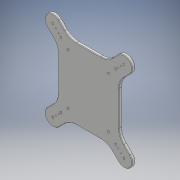
# Autodesk Inventor part: body
Saved by Autodesk Inventor 2018 (Build 220112000, 112)
## iProperties
Created: 2018-04-07
Part Number: body
Material: Generic
Document SubType Name: Modeling
Designer: Matyi
Density: 1 g/cm^3
Appearance: Default
Author: Matyi
Autodesk Inventor part; units mm, degrees
ref_plane "YZ Plane" through (0, 0, 0) normal (1, 0, 0) x (0, 1, 0)
ref_plane "XZ Plane" through (0, 0, 0) normal (0, 1, 0) x (-1, 0, 0)
ref_plane "XY Plane" through (0, 0, 0) normal (0, 0, 1) x (1, 0, 0)
sketch "Sketch1" plane through (0, 0, 0) normal (0, 1, 0) x (-1, 0, 0)
  line L0 (0, 0) -> (60, 0)
  line L1 (60, 0) -> (60, -70)
  line L2 (60, -70) -> (0, -70)
  line L3 (0, -70) -> (0, 0)
  circle A0 centre (3, -3) radius 1
  circle A1 centre (57, -3) radius 1
  circle A2 centre (57, -67) radius 1
  circle A3 centre (3, -67) radius 1
  circle A4 centre (65, 5) radius 1
  circle A5 centre (65, -75) radius 1
  circle A6 centre (-5, -75) radius 1
  circle A7 centre (-5, 5) radius 1
  arc A8 (0.6569, 10.6569) -> (-10.6569, -0.6569) centre (-5, 5) ccw
  line L4 (-5, 5) -> (0.6569, 10.6569) construction
  line L5 (-5, 5) -> (3, 5) construction
  line L6 (-5, 5) -> (-10.6569, -0.6569) construction
  arc A9 (70.6569, -0.6569) -> (59.3431, 10.6569) centre (65, 5) ccw
  line L7 (65, 5) -> (70.6569, -0.6569) construction
  line L8 (65, 5) -> (73, 5) construction
  line L9 (65, 5) -> (59.3431, 10.6569) construction
  arc A10 (59.3431, -80.6569) -> (70.6569, -69.3431) centre (65, -75) ccw
  line L10 (65, -75) -> (59.3431, -80.6569) construction
  line L11 (65, -75) -> (73, -75) construction
  line L12 (65, -75) -> (70.6569, -69.3431) construction
  arc A11 (-10.6569, -69.3431) -> (0.6569, -80.6569) centre (-5, -75) ccw
  line L13 (-5, -75) -> (0.6569, -80.6569) construction
  line L14 (-5, -75) -> (3, -75) construction
  line L15 (-5, -75) -> (-10.6569, -69.3431) construction
  line L16 (70.6569, -0.6569) -> (60, -11.3137)
  line L17 (59.3431, 10.6569) -> (48.6863, 0)
  line L18 (0.6569, 10.6569) -> (11.3137, 0)
  line L19 (-10.6569, -0.6569) -> (0, -11.3137)
  line L20 (-10.6569, -69.3431) -> (0, -58.6863)
  line L21 (0.6569, -80.6569) -> (11.3137, -70)
  line L22 (59.3431, -80.6569) -> (48.6863, -70)
  line L23 (70.6569, -69.3431) -> (60, -58.6863)
  circle A12 centre (62.1716, 2.1716) radius 0.5
  circle A13 centre (59.3431, -0.6569) radius 0.5
  line L24 (65, 5) -> (62.1716, 2.1716)
  line L25 (65, 5) -> (69, 5) construction
  line L26 (62.1716, 2.1716) -> (59.3431, -0.6569)
  line L27 (-5, 5) -> (-2.1716, 2.1716)
  line L28 (-2.1716, 2.1716) -> (0.6569, -0.6569)
  circle A14 centre (0.6569, -0.6569) radius 0.5
  circle A15 centre (-2.1716, 2.1716) radius 0.5
  line L29 (-5, -75) -> (-2.1716, -72.1716)
  line L30 (-2.1716, -72.1716) -> (0.6569, -69.3431)
  circle A16 centre (0.6569, -69.3431) radius 0.5
  circle A17 centre (-2.1716, -72.1716) radius 0.5
  line L31 (65, -75) -> (62.1716, -72.1716)
  line L32 (62.1716, -72.1716) -> (59.3431, -69.3431)
  circle A18 centre (59.3431, -69.3431) radius 0.5
  circle A19 centre (62.1716, -72.1716) radius 0.5
  circle A20 centre (50, -10) radius 1
  circle A21 centre (10, -10) radius 1
  circle A22 centre (50, -60) radius 1
  circle A23 centre (10, -60) radius 1
  dimension "d0" = 60
  dimension "d1" = 70
  dimension "d2" = 2
  dimension "d3" = 2
  dimension "d4" = 2
  dimension "d5" = 2
  dimension "d6" = 3
  dimension "d7" = 3
  dimension "d8" = 3
  dimension "d9" = 3
  dimension "d10" = 3
  dimension "d11" = 3
  dimension "d12" = 3
  dimension "d13" = 3
  dimension "d19" = 2
  dimension "d20" = 2
  dimension "d21" = 2
  dimension "d22" = 2
  dimension "d23" = 5
  dimension "d24" = 5
  dimension "d25" = 5
  dimension "d26" = 5
  dimension "d27" = 5
  dimension "d28" = 5
  dimension "d29" = 5
  dimension "d30" = 5
  dimension "d32" = 8
  dimension "d33" = 45
  dimension "d34" = 180
  dimension "d35" = 8
  dimension "d36" = 45
  dimension "d37" = 180
  dimension "d38" = 8
  dimension "d39" = 135
  dimension "d40" = 180
  dimension "d41" = 8
  dimension "d42" = 45
  dimension "d43" = 180
  dimension "d48" = 1
  dimension "d49" = 1
  dimension "d50" = 4
  dimension "d51" = 135
  dimension "d52" = 4
  dimension "d53" = 1
  dimension "d54" = 1
  dimension "d55" = 1
  dimension "d56" = 1
  dimension "d57" = 1
  dimension "d58" = 1
  dimension "d64" = 2
  dimension "d65" = 2
  dimension "d66" = 2
  dimension "d67" = 2
  dimension "d68" = 10
  dimension "d69" = 10
  dimension "d70" = 10
  dimension "d71" = 10
  dimension "d72" = 10
  dimension "d73" = 10
  dimension "d74" = 10
  dimension "d75" = 10
  constraints: 66 end point, 24 centre point, 13 point on line, 9 coincident, 9 point on circle, 6 horizontal, 5 equal length, 5 parallel, 5 perpendicular, 2 tangent
  measures "d0" distance of L1.end L2.end
  measures "d1" distance of L0.end L1.end
  measures "d2" diameter of A0
  measures "d3" diameter of A1
  measures "d4" diameter of A2
  measures "d5" diameter of A3
  measures "d6" distance from line of L3 A0.centre
  measures "d7" distance from line of L0 A0.centre
  measures "d8" distance from line of L1 A1.centre
  measures "d9" distance from line of L0 A1.centre
  measures "d10" distance from line of L2 A2.centre
  measures "d11" distance from line of L1 A2.centre
  measures "d12" distance from line of L2 A3.centre
  measures "d13" distance from line of L3 A3.centre
  measures "d19" diameter of A4
  measures "d20" diameter of A5
  measures "d21" diameter of A6
  measures "d22" diameter of A7
  measures "d23" distance from line of L1 A4.centre
  measures "d24" distance from line of L0 A4.centre
  measures "d25" distance from line of L2 A5.centre
  measures "d26" distance from line of L1 A5.centre
  measures "d27" distance from line of L2 A6.centre
  measures "d28" distance from line of L3 A6.centre
  measures "d29" distance from line of L3 A7.centre
  measures "d30" distance from line of L0 A7.centre
  measures "d32" radius of A8
  measures "d33" angle of L5 L4
  measures "d34" angle of L6 L4
  measures "d35" radius of A9
  measures "d36" angle of L7 L8
  measures "d37" angle of L9 L7
  measures "d38" radius of A10
  measures "d39" angle of L10 L11
  measures "d40" angle of L12 L10
  measures "d41" radius of A11
  measures "d42" angle of L13 L14
  measures "d43" angle of L15 L13
  measures "d48" diameter of A12
  measures "d49" diameter of A13
  measures "d50" distance of L7.start L24.end
  measures "d51" angle of L24 L25
  measures "d52" distance of L24.end L26.end
  measures "d53" diameter of A14
  measures "d54" diameter of A15
  measures "d55" diameter of A16
  measures "d56" diameter of A17
  measures "d57" diameter of A18
  measures "d58" diameter of A19
  measures "d64" diameter of A20
  measures "d65" diameter of A21
  measures "d66" diameter of A22
  measures "d67" diameter of A23
  measures "d68" distance from line of L0 A21.centre
  measures "d69" distance from line of L3 A21.centre
  measures "d70" distance from line of L0 A20.centre
  measures "d71" distance from line of L1 A20.centre
  measures "d72" distance from line of L1 A22.centre
  measures "d73" distance from line of L2 A22.centre
  measures "d74" distance from line of L3 A23.centre
  measures "d75" distance from line of L2 A23.centre
extrude "Extrusion4" add sketch "Sketch1" along normal blind 3
fillet "Fillet6" radius 16 8 edges at (-60, 1.5, -11.3137) (-11.3137, 1.5, -70) (-60, 1.5, -58.6863) (-11.3137, 1.5, 0) (-48.6863, 1.5, -70) (0, 1.5, -11.3137) (-48.6863, 1.5, 0) (0, 1.5, -58.6863)
fillet "Fillet7" radius 0.5 32 edges at (7.6716, 0, -66.3579) (10.6569, 0, -80.6569) (-3.6421, 0, -77.6716) (-30, 0, -70) (-56.3579, 0, -77.6716) (-70.6569, 0, -80.6569) (-67.6716, 0, -66.3579) (-60, 0, -35) (-67.6716, 0, -3.6421) (-70.6569, 0, 10.6569) (-56.3579, 0, 7.6716) (-30, 0, 0) (-3.6421, 0, 7.6716) (10.6569, 0, 10.6569) (7.6716, 0, -3.6421) (0, 0, -35) (7.6716, 3, -66.3579) (10.6569, 3, -80.6569) (-3.6421, 3, -77.6716) (-30, 3, -70) (-56.3579, 3, -77.6716) (-70.6569, 3, -80.6569) (-67.6716, 3, -66.3579) (-60, 3, -35) (-67.6716, 3, -3.6421) (-70.6569, 3, 10.6569) (-56.3579, 3, 7.6716) (-30, 3, 0) (-3.6421, 3, 7.6716) (10.6569, 3, 10.6569) (7.6716, 3, -3.6421) (0, 3, -35)
body "Solid4"
